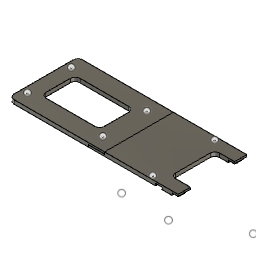
Awesome Spooler Mount (Autodesk Fusion 360 design; units mm, degrees)
Autodesk Fusion 360 part; units mm, degrees
note: some values were not read from the file. Set by a fixed rule: which sketch regions a step uses.
sketch "Sketch1" plane through (0, 0, 0) normal (0, 0, 1) x (1, 0, 0)
  line L0 (240.5, -70.5) -> (-250.5, -70.5) construction
  line L1 (-250.5, -70.5) -> (-250.5, 60.5) construction
  line L2 (-250.5, 70.5) -> (250.5, 70.5) construction
  line L3 (250.5, 70.5) -> (250.5, -60.5) construction
  line L4 (250.5, -70.5) -> (-250.5, 70.5) construction
  line L5 (-250.5, -70.5) -> (250.5, 70.5) construction
  line L6 (240.5, 70.5) -> (-70.5, 70.5)
  line L7 (30.5, 70.5) -> (30.5, -70.5)
  line L8 (117, -70.5) -> (240.5, -70.5)
  line L9 (250.5, -60.5) -> (250.5, 60.5)
  arc A0 (240.5, -70.5) -> (250.5, -60.5) centre (240.5, -60.5) ccw construction
  arc A1 (240.5, -70.5) -> (250.5, -60.5) centre (240.5, -60.5) ccw
  arc A2 (250.5, 60.5) -> (240.5, 70.5) centre (240.5, 60.5) ccw
  line L10 (140, 70.5) -> (140, -70.5) construction
  line L11 (250.5, 0) -> (30.5, 0) construction
  line L12 (55.5, 35.5) -> (55.5, -35.1)
  line L13 (65.5, -45.1) -> (215.5, -45.1)
  line L14 (225.5, -35.1) -> (225.5, 35.5)
  line L15 (215.5, 45.5) -> (65.5, 45.5)
  arc A3 (65.5, 45.5) -> (55.5, 35.5) centre (65.5, 35.5) ccw
  arc A4 (55.5, -35.1) -> (65.5, -45.1) centre (65.5, -35.1) ccw
  arc A5 (225.5, 35.5) -> (215.5, 45.5) centre (215.5, 35.5) ccw
  arc A6 (215.5, -45.1) -> (225.5, -35.1) centre (215.5, -35.1) ccw
  line L16 (28, -170) -> (28, -40) construction
  line L17 (0, -118.25) -> (155.4243, -118.25) construction
  line L18 (63, -70.5) -> (104, -70.5)
  line L19 (129, -70.5) -> (129, -135.5)
  line L20 (114, -150.5) -> (38, -150.5)
  line L21 (23, -135.5) -> (23, -70.5)
  line L22 (-83.5, 130) -> (-83.5, -190) construction
  line L23 (83.5, -64.0302) -> (83.5, -190) construction
  line L24 (-240.5, 70.5) -> (-70.5, 70.5)
  line L25 (-70.5, -70.5) -> (-240.5, -70.5)
  line L26 (-250.5, -60.5) -> (-250.5, 70.5)
  line L27 (-220.6, 25) -> (-220.6, -25)
  line L28 (-210.6, -35) -> (-110.4, -35)
  line L29 (-100.4, -25) -> (-100.4, 25)
  line L30 (-110.4, 35) -> (-210.6, 35)
  arc A7 (-240.5, 70.5) -> (-250.5, 60.5) centre (-240.5, 60.5) ccw
  arc A8 (-250.5, -60.5) -> (-240.5, -70.5) centre (-240.5, -60.5) ccw
  arc A9 (-210.6, 35) -> (-220.6, 25) centre (-210.6, 25) ccw
  arc A10 (-220.6, -25) -> (-210.6, -35) centre (-210.6, -25) ccw
  arc A11 (-100.4, 25) -> (-110.4, 35) centre (-110.4, 25) ccw
  arc A12 (-110.4, -35) -> (-100.4, -25) centre (-110.4, -25) ccw
  arc A13 (23, -135.5) -> (38, -150.5) centre (38, -135.5) ccw
  arc A14 (114, -150.5) -> (129, -135.5) centre (114, -135.5) ccw
  line L31 (-72.5, -5) -> (-80.5, -5)
  line L32 (-80.5, 5.0637) -> (-72.5, 5.0637)
  arc A15 (-70.5, -15) -> (-59.5, -15) centre (-65, -15) ccw
  line L33 (-59.5, -15) -> (-59.5, 15)
  arc A16 (-59.5, 15) -> (-70.5, 15) centre (-65, 15) ccw
  line L34 (-65, 15) -> (-65, -15) construction
  line L35 (-70.5, 70.5) -> (-70.5, 7.0637)
  line L36 (-70.5, -7) -> (-70.5, -70.5)
  line L37 (-70.5, 15) -> (-70.5, 7.0637)
  line L38 (-70.5, -7) -> (-70.5, -15)
  arc A17 (-72.5, 5.0637) -> (-70.5, 7.0637) centre (-72.5, 7.0637) ccw
  arc A18 (-70.5, -7) -> (-72.5, -5) centre (-72.5, -7) ccw
  line L39 (-88, 8.0637) -> (-88, 70.5)
  line L40 (-88, -8) -> (-88, -70.5)
  line L41 (78, -57.8) -> (89, -57.8) construction
  line L42 (-54.8367, -70.5) -> (-54.8367, 70.5)
  line L43 (87.3815, -51.1) -> (87.3815, -51.9884)
  arc A19 (87.3815, -64.5) -> (92.6185, -64.5) centre (90, -64.5) ccw
  line L44 (92.6185, -64.5) -> (92.6185, -51.1)
  arc A20 (92.6185, -51.1) -> (87.3815, -51.1) centre (90, -51.1) ccw
  line L45 (90, -51.1) -> (90, -64.5) construction
  line L46 (84.5, -52.9884) -> (86.3815, -52.9884)
  line L47 (84.5, -63.0302) -> (86.3815, -63.0302)
  line L48 (83.5, -70.5) -> (83.5, -45.1)
  arc A21 (83.5, -51.9884) -> (84.5, -52.9884) centre (84.5, -51.9884) ccw
  arc A22 (84.5, -63.0302) -> (83.5, -64.0302) centre (84.5, -64.0302) ccw
  arc A23 (86.3815, -52.9884) -> (87.3815, -51.9884) centre (86.3815, -51.9884) ccw
  line L49 (87.3815, -64.0302) -> (87.3815, -64.5)
  arc A24 (87.3815, -64.0302) -> (86.3815, -63.0302) centre (86.3815, -64.0302) ccw
  line L50 (95.9753, -45.1) -> (95.9753, -70.5)
  line L51 (83.5, 70.5) -> (83.5, 45.5)
  arc A25 (84.5, 52.9884) -> (83.5, 51.9884) centre (84.5, 51.9884) ccw
  line L52 (84.5, 52.9884) -> (86.3815, 52.9884)
  arc A26 (87.3815, 51.9884) -> (86.3815, 52.9884) centre (86.3815, 51.9884) ccw
  line L53 (87.3815, 51.1) -> (87.3815, 51.9884)
  arc A27 (87.3815, 51.1) -> (92.6185, 51.1) centre (90, 51.1) ccw
  line L54 (92.6185, 64.5) -> (92.6185, 51.1)
  arc A28 (92.6185, 64.5) -> (87.3815, 64.5) centre (90, 64.5) ccw
  line L55 (87.3815, 64.0302) -> (87.3815, 64.5)
  arc A29 (86.3815, 63.0302) -> (87.3815, 64.0302) centre (86.3815, 64.0302) ccw
  line L56 (84.5, 63.0302) -> (86.3815, 63.0302)
  arc A30 (83.5, 64.0302) -> (84.5, 63.0302) centre (84.5, 64.0302) ccw
  line L57 (95.9753, 45.5) -> (95.9753, 70.5)
  line L58 (47, -66) -> (49, -66)
  arc A31 (65, -66) -> (65, -60) centre (65, -63) ccw
  line L59 (65, -60) -> (47, -60)
  arc A32 (47, -60) -> (47, -66) centre (47, -63) ccw
  line L60 (47, -63) -> (65, -63) construction
  line L61 (102.1654, -66) -> (104, -66)
  arc A33 (119, -66) -> (119, -60.0603) centre (119, -63.0302) ccw
  line L62 (119, -60.0603) -> (102.1654, -60.0603)
  arc A34 (102.1654, -60.0603) -> (102.1654, -66) centre (102.1654, -63.0302) ccw
  line L63 (102.1654, -63.0302) -> (119, -63.0302) construction
  line L64 (50, -67) -> (50, -69.5)
  line L65 (62, -67) -> (62, -69.5)
  line L66 (105, -67) -> (105, -69.5)
  line L67 (116, -67) -> (116, -69.5)
  arc A35 (105, -67) -> (104, -66) centre (104, -67) ccw
  line L68 (117, -66) -> (119, -66)
  arc A36 (117, -66) -> (116, -67) centre (117, -67) ccw
  line L69 (23, -70.5) -> (49, -70.5)
  arc A37 (50, -67) -> (49, -66) centre (49, -67) ccw
  line L70 (63, -66) -> (65, -66)
  arc A38 (63, -66) -> (62, -67) centre (63, -67) ccw
  arc A39 (49, -70.5) -> (50, -69.5) centre (49, -69.5) ccw
  arc A40 (62, -69.5) -> (63, -70.5) centre (63, -69.5) ccw
  arc A41 (104, -70.5) -> (105, -69.5) centre (104, -69.5) ccw
  line L71 (129, -70.5) -> (116, -70.5029)
  arc A42 (116, -69.5) -> (117, -70.5) centre (117, -69.5) ccw
  line L72 (49, -70.5) -> (63, -70.5)
  line L73 (104, -70.5) -> (117, -70.5)
  line L74 (-70.5, -70.5) -> (30.5, -70.5)
  line L75 (-80.5, 5.0637) -> (-85, 5.0637)
  line L76 (-80.5, -5) -> (-85, -5)
  arc A43 (-85, -5) -> (-88, -8) centre (-85, -8) ccw
  arc A44 (-88, 8.0637) -> (-85, 5.0637) centre (-85, 8.0637) ccw
  line L77 (-88, 8.0637) -> (-88, -8)
  point P0 (250.5, -70.5)
  point P1 (37.5, -63.5)
  point P2 (37.5, 63.5)
  point P3 (243.5, 63.5)
  point P4 (243.5, -63.5)
  point P5 (28, -118.25)
  point P6 (23, -150.5)
  point P7 (124, -118.25)
  point P8 (-250.5, -70.5)
  point P9 (-237.8, 45.2)
  point P10 (-237.8, -44.795)
  point P11 (-83.5, -44.795)
  point P12 (-83.5, 45.2)
  dimension "d1" = 501
  dimension "d2" = 141
  dimension "d3" = 220
  dimension "d4" = 141
  dimension "d9" = 10
  dimension "d12" = 7
  dimension "d13" = 7
  dimension "d14" = 7
  dimension "d15" = 7
  dimension "d16" = 7
  dimension "d17" = 7
  dimension "d18" = 7
  dimension "d19" = 7
  dimension "d23" = 25
  dimension "d24" = 25
  dimension "d25" = 25
  dimension "d26" = 25.4
  dimension "d27" = 10
  dimension "d28" = 10
  dimension "d29" = 10
  dimension "d30" = 10
  dimension "d32" = 54.75
  dimension "d33" = 106
  dimension "d34" = 80
  dimension "d35" = 5
  dimension "d36" = 96
  dimension "d37" = 167
  dimension "d38" = 167
  dimension "d39" = 180
  dimension "d40" = 141
  dimension "d41" = 35.5
  dimension "d42" = 35.5
  dimension "d43" = 29.9
  dimension "d44" = 29.9
  dimension "d45" = 10
  dimension "d46" = 10
  dimension "d47" = 10
  dimension "d48" = 10
  dimension "d49" = 10
  dimension "d50" = 25.3
  dimension "d51" = 12.7
  dimension "d52" = 25.705
  dimension "d53" = 13
  dimension "d54" = 25.3
  dimension "d55" = 15
  dimension "d56" = 2
  dimension "d59" = 12.7
  dimension "d60" = 1
  dimension "d61" = 1
  dimension "d62" = 1
  dimension "d63" = 1
  dimension "d64" = 1
  dimension "d65" = 1
  dimension "d66" = 1
  dimension "d77" = 6
  dimension "d78" = 6
  dimension "d119" = 3
  dimension "d120" = 3
  dimension "d121" = 25.705
  dimension "d122" = 12.7
  constraint horizontal L0
  constraint perpendicular L0 L1
  constraint parallel L0 L2
  constraint parallel L1 L3
  constraint coincident L4 origin
  constraint coincident L5 origin
  constraint horizontal L6
  constraint vertical L7
  constraint horizontal L8
  constraint vertical L9
  constraint coincident P0 L3
  constraint coincident P0 L0
  constraint tangent L3 A0
  constraint tangent L0 A0
  constraint coincident P0 L9
  constraint coincident P0 L8
  constraint tangent L9 A1
  constraint tangent L8 A1
  constraint equal A0 A1
  constraint coincident L2.end L6
  constraint coincident L2.end L9
  constraint tangent L6 A2
  constraint tangent L9 A2
  constraint equal A0 A2
  constraint midpoint L9 L11.start
  constraint perpendicular L11 L12
  constraint perpendicular L10 L13
  constraint perpendicular L11 L14
  constraint perpendicular L14 L15
  constraint tangent L12 A3
  constraint tangent L15 A3
  constraint tangent L12 A4
  constraint tangent L13 A4
  constraint tangent L15 A5
  constraint tangent L14 A5
  constraint tangent L13 A6
  constraint tangent L14 A6
  constraint perpendicular L0 L16
  constraint perpendicular L16 L17
  constraint coincident L17 P5
  constraint coincident L16 P5
  constraint horizontal L18
  constraint vertical L19
  constraint horizontal L20
  constraint vertical L21
  constraint coincident L0 L21.end
  constraint coincident L17 P7
  constraint coincident L7 L11.end
  constraint coincident L6 L10.start
  constraint coincident L0 L7.end
  constraint coincident L8 L10.end
  constraint vertical L22
  constraint perpendicular L20 L23
  constraint horizontal L24
  constraint vertical L35
  constraint horizontal L25
  constraint vertical L26
  constraint perpendicular L0 L27
  constraint perpendicular L3 L28
  constraint perpendicular L0 L29
  constraint perpendicular L29 L30
  constraint coincident L2.start L1
  constraint coincident L2.start L24
  constraint tangent L1 A7
  constraint tangent L24 A7
  constraint coincident P8 L26
  constraint coincident P8 L25
  constraint tangent L26 A8
  constraint tangent L25 A8
  constraint tangent L27 A9
  constraint tangent L30 A9
  constraint tangent L27 A10
  constraint tangent L28 A10
  constraint tangent L30 A11
  constraint tangent L29 A11
  constraint tangent L28 A12
  constraint tangent L29 A12
  constraint equal A11 A12
  constraint coincident P6 L21
  constraint coincident P6 L20
  constraint tangent L21 A13
  constraint tangent L20 A13
  constraint tangent L19 A14
  constraint tangent L20 A14
  constraint equal A13 A14
  constraint perpendicular L8 L35
  constraint perpendicular L22 L31
  constraint perpendicular L32 L35
  constraint tangent A15 L37
  constraint tangent A15 L33
  constraint parallel L33 L37
  constraint tangent L33 A16
  constraint tangent A16 L37
  constraint parallel L34 L35
  constraint collinear L35 L36
  constraint collinear L37 L38
  constraint tangent L32 A17
  constraint tangent L37 A17
  constraint tangent L31 A18
  constraint tangent L36 A18
  constraint equal A17 A18
  constraint perpendicular L10 L41
  constraint perpendicular L6 L42
  constraint tangent L43 A19
  constraint tangent A19 L44
  constraint parallel L43 L44
  constraint tangent L44 A20
  constraint tangent L43 A20
  constraint perpendicular L41 L45
  constraint perpendicular L43 L46
  constraint perpendicular L43 L47
  constraint coincident L13 L48.end
  constraint coincident L23 L48.end
  constraint coincident L18 L48.start
  constraint coincident L23 L48.start
  constraint tangent L48 A21
  constraint tangent L46 A21
  constraint tangent L47 A22
  constraint tangent L23 A22
  constraint equal A21 A22
  constraint coincident A19.start L43
  constraint tangent L46 A23
  constraint tangent L43 A23
  constraint equal A21 A23
  constraint tangent A19 L49
  constraint tangent L47 A24
  constraint tangent L49 A24
  constraint coincident L13 L50.start
  constraint coincident L18 L50.end
  constraint symmetric L11 L43.start L53.start
  constraint symmetric L11 A19.start A28.end
  constraint symmetric L11 A19.end L54.start
  constraint symmetric L11 L44.end A27.end
  constraint symmetric L11 A19 A28
  constraint symmetric L11 A20 A27
  constraint symmetric L11 L48.start L51.start
  constraint symmetric L11 A21.start A25.end
  constraint symmetric L11 L46.start A25.start
  constraint symmetric L11 A21 A25
  constraint symmetric L11 L47.start L56.start
  constraint symmetric L11 L23.start A30.start
  constraint symmetric L11 A22 A30
  constraint symmetric L11 L46.end L52.end
  constraint symmetric L11 L43.end A26.start
  constraint symmetric L11 A23 A26
  constraint symmetric L11 L47.end A29.start
  constraint symmetric L11 L49.start L55.start
  constraint symmetric L11 A24 A29
  constraint symmetric L11 L50.end L57.end
  constraint coincident L15 L57.start
  constraint perpendicular L15 L57
  constraint vertical L51
  constraint tangent L58 A31
  constraint tangent A31 L59
  constraint parallel L58 L59
  constraint tangent L59 A32
  constraint tangent L58 A32
  constraint parallel L18 L60
  constraint tangent L61 A33
  constraint tangent A33 L62
  constraint parallel L61 L62
  constraint tangent L62 A34
  constraint tangent L61 A34
  constraint perpendicular L50 L63
  constraint vertical L64
  constraint vertical L65
  constraint vertical L66
  constraint vertical L67
  constraint coincident A33.start L61
  constraint tangent L66 A35
  constraint tangent L61 A35
  constraint tangent A33 L68
  constraint tangent L67 A36
  constraint tangent L68 A36
  constraint coincident A31.start L58
  constraint tangent L58 A37
  constraint tangent L64 A37
  constraint tangent A31 L70
  constraint tangent L65 A38
  constraint tangent L70 A38
  constraint coincident L19.start L69
  constraint tangent L64 A39
  constraint tangent L69 A39
  constraint equal A38 A39
  constraint coincident L21.end L18
  constraint tangent L65 A40
  constraint tangent L18 A40
  constraint equal A38 A40
  constraint coincident L19.start L18
  constraint tangent L66 A41
  constraint tangent L18 A41
  constraint equal A38 A41
  constraint coincident L71.end L67
  constraint tangent L67 A42
  constraint tangent L8 A42
  constraint perpendicular L22 L76
  constraint tangent L76 A43
  constraint coincident L40.start A43.end
  constraint tangent L75 A44
  constraint tangent L39 A44
  constraint tangent A43 L77
  measures "d1" distance of L2.start L2.end
  measures "d2" distance of P8 L2.start
  measures "d3" distance of L2.end L7.start
  measures "d4" distance of L2.end P0
  measures "d9" radius of A0
  measures "d12" distance of L7 P1
  measures "d13" distance of L8 P1
  measures "d14" distance of L6 P2
  measures "d15" distance of L7 P2
  measures "d16" distance of L9 P3
  measures "d17" distance of L6 P3
  measures "d18" distance of L3 P4
  measures "d19" distance of L8 P4
  measures "d23" distance of L7 L12
  measures "d24" distance of L6 L15
  measures "d25" distance of L9 L14
  measures "d26" distance of L8 L13
  measures "d27" radius of A3
  measures "d28" radius of A4
  measures "d29" radius of A5
  measures "d30" radius of A6
  measures "d32" distance of P1 L17
  measures "d33" distance of L21.end L19.start
  measures "d34" distance of L21.end P6
  measures "d35" distance of P5 L21
  measures "d36" distance of P5 P7
  measures "d37" distance of L1 L22
  measures "d38" distance of L3 L23
  measures "d39" distance of L2.start L6.end
  measures "d40" distance of L2.start P8
  measures "d41" distance of L2 L30
  measures "d42" distance of L0 L28
  measures "d43" distance of L26 L27
  measures "d44" distance of L29 L35
  measures "d45" radius of A7
  measures "d46" radius of A8
  measures "d47" radius of A9
  measures "d48" radius of A10
  measures "d49" radius of A11
  measures "d50" distance of L2 P9
  measures "d51" distance of L26 P9
  measures "d52" distance of L0 P10
  measures "d53" distance of P11 L35
  measures "d54" distance of L24 P12
  measures "d55" radius of A13
  measures "d56" radius of A17
  measures "d59" distance of L0 L41
  measures "d60" radius of A21
  measures "d61" radius of A24
  measures "d62" radius of A35
  measures "d63" radius of A36
  measures "d64" radius of A37
  measures "d65" radius of A38
  measures "d66" radius of A42
  measures "d77" distance of L13 A20.centre
  measures "d78" distance of L18 A19.centre
  measures "d119" radius of A43
  measures "d120" radius of A44
  measures "d121" distance of L25 P11
  measures "d122" distance of L26 P10
extrude "Extrude4" add sketch "Sketch1" along normal blind 8 contours L6 L8 L9 A1 A2 L13 L14 L15 A5 A6 L18 L50 L57 L61 A33 L62 A34 L66 L67 A35 L68 A36 A41 A42 makes body 1
extrude "Extrude5" add sketch "Sketch1" along normal blind 8 separate body contours L6 L7 L12 L13 L15 A3 A4 L18 L48 L51 L58 A31 L59 A32 L64 L65 L69 A37 L70 A38 A39 A40 | L6 L7 L42 L69 L74 | L51 A25 L52 A26 L53 A27 L54 A28 L55 A29 L56 A30 | L43 A19 L44 A20 L46 L47 L48 A21 A22 A23 L49 A24 makes body 2
extrude "Extrude6" add sketch "Sketch1" along normal blind 8 separate body contours L24 L25 L26 A7 A8 L39 L40 L77 | L31 L32 A15 L33 A16 L35 L36 L37 L38 A17 A18 L75 L76 A43 A44 L77 makes body 3
extrude "Extrude7" add sketch "Sketch1" along normal blind 4 separate body contours L6 A15 L33 A16 L35 L36 L42 L74 | L24 L32 L35 L37 A17 L39 L75 A44 | L25 L31 L36 L38 A18 L40 L76 A43 makes body 4
combine "Combine4" operation add target body 2 tool bodies 4
extrude "Extrude8" add sketch "Sketch1" along normal blind 4 separate body contours L6 L15 L51 A25 L52 A26 L53 A27 L54 A28 L55 A29 L56 A30 L57 | L13 L18 L43 A19 L44 A20 L46 L47 L48 A21 A22 A23 L49 A24 L50 makes body 5 at (94.8563, 60.1667, 0) makes body 6 at (94.8563, -60.0333, 0)
combine "Combine5" operation add target body 1 tool bodies 5 6
extrude "Extrude9" add sketch "Sketch1" against normal blind 3.6 from surface at 8 contours L6 L15 L51 A25 L52 A26 L53 A27 L54 A28 L55 A29 L56 A30 L57 | L58 A31 L59 A32 L64 L65 A37 L70 A38 A39 A40 L72 | L13 L18 L43 A19 L44 A20 L46 L47 L48 A21 A22 A23 L49 A24 L50 bodies 2
extrude "Extrude10" add sketch "Sketch1" against normal blind 3.6 from surface at 8 contours L61 A33 L62 A34 L66 L67 A35 L68 A36 A41 A42 L73 bodies 1
extrude "Extrude11" add sketch "Sketch1" against normal blind 3.6 from surface at 8 contours L6 A15 L33 A16 L35 L36 L42 L74 | L24 L32 L35 L37 A17 L39 L75 A44 | L25 L31 L36 L38 A18 L40 L76 A43 bodies 3
extrude "Extrude12" add sketch "Sketch1" along normal blind 8 separate body contours L8 L18 L19 L20 L21 A13 A14 L69 L72 L73 L74 makes body 7
extrude "Extrude13" add sketch "Sketch1" along normal blind 4 contours L58 A31 L59 A32 L64 L65 A37 L70 A38 A39 A40 L72 | L61 A33 L62 A34 L66 L67 A35 L68 A36 A41 A42 L73 bodies 7
ref_plane "WorkPlane1" through (20.5693, 0, 8) normal (0, 0, 1) x (1, 0, 0)
sketch "Sketch3" plane through (20.5693, 0, 8) normal (0, 0, 1) x (1, 0, 0)
  point P0 (7.4307, -118.25)
  point P1 (103.4346, -118.25)
  point P2 (222.5, 63.5)
  point P3 (222.5, -63.5)
  point P4 (16.5, 63.5)
  point P5 (-259.3, -44.7954)
  point P6 (-259.3, 45.2)
  point P7 (-104.5, 45.2)
  point P8 (-104.5, -44.7954)
  point P9 (16.5, -63.5)
hole "Hole2" at (-238.7307, 45.2, 8) at (-83.9307, 45.2, 8) at (37.0693, 63.5, 8) at (243.0693, 63.5, 8) at (243.0693, -63.5, 8) at (37.0693, -63.5, 8) at (-83.9307, -44.7954, 8) at (-238.7307, -44.7954, 8) direction (0, 0, -1) diameter 2.9 depth 8 tip angle 180 countersink diameter 3.19 countersink angle 70 bodies 1 2 3
hole "Hole1" [rolled back] hole depth 8 hole diameter 2.9 tip angle 180 csdiameter 3.19 csangle 70
move_face "OffsetFaces2" [rolled back]
hidden bodies 1 7
equation "d3 = mainwidth"
equation "d4 = mainheight"
equation "outsideframeradius = 10 mm"
equation "insideframeradius = 10 mm"
equation "d9 = outsideframeradius"
equation "mainholedistance = 7 mm"
equation "d12 = mainholedistance"
equation "mainwidth = 220 mm"
equation "mainheight = 141 mm"
equation "mainborderwidth = 25 mm"
equation "d23 = mainborderwidth"
equation "d24 = mainborderwidth"
equation "d25 = mainborderwidth"
equation "d26 = mainborderwidth + 0.4 mm"
equation "d27 = insideframeradius"
equation "d28 = insideframeradius"
equation "d29 = insideframeradius"
equation "d30 = insideframeradius"
equation "d45 = outsideframeradius"
equation "d46 = outsideframeradius"
equation "d47 = insideframeradius"
equation "d48 = insideframeradius"
equation "d49 = insideframeradius"
equation "mountthickness = 8 mm"
equation "slotOffset = mountthickness / 2"
equation "slotGap = 0.4 mm"
equation "d83 = mountthickness"
equation "d85 = mountthickness"
equation "d87 = mountthickness"
equation "d89 = slotOffset"
equation "d91 = slotOffset"
equation "d94 = -slotOffset + slotGap"
equation "d97 = -slotOffset + slotGap"
equation "d100 = -slotOffset + slotGap"
equation "d102 = mountthickness"
equation "d104 = slotOffset"
equation "d107 = mountthickness"
equation "matingTolerance = 0.1 mm"
equation "d113 = -matingTolerance"
named bodies: "Spooler Mount Right", "Spooler Mount Middle", "Spooler Mount Left", "Spooler Motor Mount"
